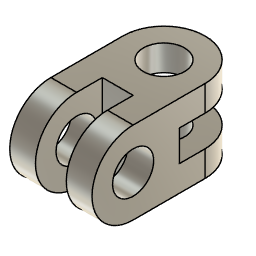
25 (Autodesk Fusion 360 design; units mm, degrees)
Autodesk Fusion 360 part; units mm, degrees
sketch "草图1" plane through (0, 0, 0) normal (0, 0, 1) x (1, 0, 0)
  circle A0 centre (0, 22) radius 4
  circle A1 centre (0, 22) radius 8
  line L0 (-8, 22) -> (-8, 0)
  line L1 (-8, 0) -> (8, 0)
  line L2 (8, 0) -> (8, 22)
  line L3 (0, 108.3744) -> (0, -35) construction
  dimension "d1" = 8
  dimension "d2" = 16
  dimension "d3" = 22
  constraint concentric A0 A1
  constraint coincident A1 L0.start
  constraint vertical L0
  constraint perpendicular L0 L1
  constraint coincident A1 L2.end
  constraint tangent A1 L2
  constraint perpendicular L1 L3
  constraint collinear A0.centre L3.start L3.end
  constraint perpendicular L1 L2
  constraint tangent A1 L0
  constraint collinear origin L0.end L1.end
  measures "d1" diameter of A0
  measures "d2" diameter of A1
  measures "d3" distance of A0.centre L1
extrude "拉伸1" add sketch "草图1" along normal mid plane 16
sketch "草图2" plane through (8, 0, 0) normal (1, 0, 0) x (0, 1, 0)
  line L0 (22, -8) -> (22, 8)
  line L1 (22, 8) -> (0, 8)
  line L2 (0, 8) -> (0, -8)
  line L3 (0, -8) -> (22, -8)
  circle A0 centre (8, 0) radius 8
  circle A1 centre (8, 0) radius 4
  line L4 (8, 8) -> (22, 8)
  line L5 (22, 8) -> (22, -8)
  line L6 (8, -8) -> (22, -8)
  line L7 (-6, 0) -> (34.5187, 0) construction
  dimension "d6" = 16
  dimension "d7" = 8
  dimension "d8" = 14
  constraint concentric A0 A1
  constraint coincident A0 L4.start
  constraint coincident L0.end L1.start
  constraint coincident L0.start L3.end
  constraint coincident A0 L6.start
  constraint horizontal L7
  constraint tangent A0 L4
  constraint tangent A0 L6
  constraint collinear A0.centre L7.start L7.end
  measures "d6" diameter of A0
  measures "d7" diameter of A1
  measures "d8" distance of A0.centre L5
extrude "拉伸2" cut sketch "草图2" against normal blind 52 contours L2 L3 A0 | L1 L2 A0 | A1
sketch "草图3" plane through (8, 0, 0) normal (1, 0, 0) x (0, 1, 0)
  circle A0 centre (8, 0) radius 4
  arc A1 (8, 8) -> (8, -8) centre (8, 0) ccw
  line L0 (8, -8) -> (22, -8)
  line L1 (22, -8) -> (22, 8)
  line L2 (22, 8) -> (8, 8)
  line L3 (17, 3) -> (30, 3)
  line L4 (30, 3) -> (30, -3)
  line L5 (30, -3) -> (17, -3)
  line L6 (17, -3) -> (17, 3)
  line L7 (-4, 0) -> (38.4958, 0) construction
  line L8 (30, 8) -> (30, -8) construction
  dimension "d11" = 6
  dimension "d12" = 13
  constraint horizontal L3
  constraint vertical L4
  constraint horizontal L5
  constraint vertical L6
  constraint perpendicular L6 L7
  constraint symmetric L3 L5 L7
  constraint vertical L8
  constraint collinear L4 L8
  measures "d11" distance of L3.end L4.end
  measures "d12" horizontal distance of L3.start L8.start
extrude "拉伸3" cut sketch "草图3" against normal blind 21 contours L1 L3 L4 L5 | L1 L3 L5 L6
sketch "草图4" plane through (0, 0, 8) normal (0, 0, 1) x (-1, 0, 0)
  line L0 (8, -8) -> (-8, -8)
  line L1 (-8, -8) -> (-8, -22)
  arc A0 (-8, -22) -> (8, -22) centre (0, -22) ccw
  line L2 (8, -22) -> (8, -8)
  circle A1 centre (0, -22) radius 4
  line L3 (-3, 0) -> (3, 0)
  line L4 (3, 0) -> (3, -13)
  line L5 (3, -13) -> (-3, -13)
  line L6 (-3, -13) -> (-3, 0)
  line L7 (0, 5) -> (0, -37) construction
  line L8 (-8, 0) -> (8, 0) construction
  dimension "d15" = 6
  dimension "d16" = 13
  constraint horizontal L3
  constraint vertical L4
  constraint horizontal L5
  constraint vertical L6
  constraint perpendicular L5 L7
  constraint symmetric L4 L6 L7
  constraint perpendicular L7 L8
  measures "d15" distance of L3.start L3.end
  measures "d16" distance of L4.end L8
extrude "拉伸4" cut sketch "草图4" against normal blind 68 contours L0 L4 L5 L6 | L0 L3 L4 L6
